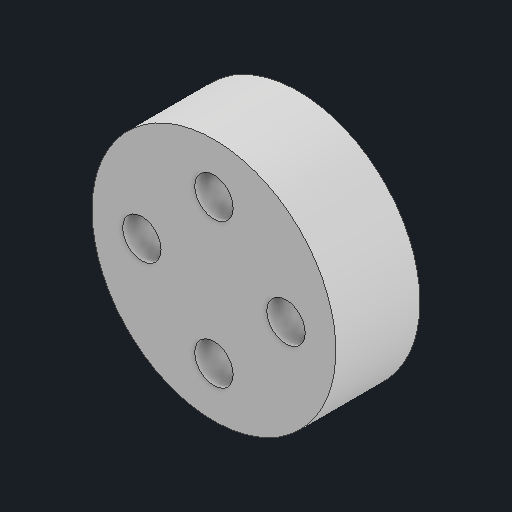
# Autodesk Inventor part: Test_ShaftB
Saved by Autodesk Inventor 2025.1 (Build 291241020, 241B)
## iProperties
Created: 2025-07-24
Part Number: Test_ShaftB
Material: 일반
Document SubType Name: Modeling
Designer: acalo
Density: 1 g/cm^3
Appearance: 기본값
Author: acalo
Autodesk Inventor part; units mm, degrees
ref_plane "YZ Plane" through (0, 0, 0) normal (1, 0, 0) x (0, 1, 0)
ref_plane "XZ Plane" through (0, 0, 0) normal (0, 1, 0) x (-1, 0, 0)
ref_plane "XY Plane" through (0, 0, 0) normal (0, 0, 1) x (1, 0, 0)
sketch "스케치1" plane through (0, 0, 0) normal (0, 0, 1) x (1, 0, 0)
  circle A0 centre (0, 0) radius 10.15
  line L0 (0, 0) -> (-6, 0)
  circle A1 centre (-6, 0) radius 1.6
  line L1 (0, 0) -> (0, 6)
  circle A2 centre (0, 6) radius 1.6
  line L2 (0, 0) -> (0, -6)
  circle A3 centre (0, -6) radius 1.6
  line L3 (0, 0) -> (6, 0)
  circle A4 centre (6, 0) radius 1.6
  dimension "d2" = 6
  dimension "d3" = 3.2
  dimension "d7" = 6
  dimension "d8" = 3.2
  dimension "d9" = 6
  dimension "d10" = 3.2
  dimension "d11" = 6
  dimension "d12" = 3.2
  dimension "d13" = 20.3
  constraints: 8 end point, 5 centre point, 5 coincident, 2 horizontal, 2 vertical
  measures "d2" distance of L0.start L0.end
  measures "d3" diameter of A1
  measures "d7" distance of L0.start L1.end
  measures "d8" diameter of A2
  measures "d9" distance of L0.start L2.end
  measures "d10" diameter of A3
  measures "d11" distance of L0.start L3.end
  measures "d12" diameter of A4
  measures "d13" diameter of A0
extrude "돌출1" add sketch "스케치1" along normal blind 6
thicken "두껍게 하기1" operation add thickness 1 both sides no extend neighbours no toward (0, 0, 1) faces at (-0.0643, -1.4706, 6)
equation "\"d5\" = d7"
